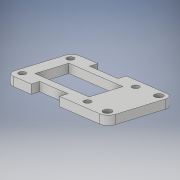
# Autodesk Inventor part: 板子6
Saved by Autodesk Inventor 2017 (Build 210142000, 142)
## iProperties
Part Number: 板子6
Material: 一般
Document SubType Name: Modeling
Designer: User
Density: 1 g/cm^3
Appearance: 預設
Author: User
Autodesk Inventor part; units mm, degrees
ref_plane "YZ Plane" through (0, 0, 0) normal (1, 0, 0) x (0, 1, 0)
ref_plane "XZ Plane" through (0, 0, 0) normal (0, 1, 0) x (-1, 0, 0)
ref_plane "XY Plane" through (0, 0, 0) normal (0, 0, 1) x (1, 0, 0)
sketch "草圖1" plane through (0, 0, 0) normal (0, 1, 0) x (-1, 0, 0)
  line L0 (-21.25, 11.85) -> (-21.25, -11.85)
  line L1 (-21.25, -11.85) -> (21.25, -11.85)
  line L2 (21.25, -11.85) -> (21.25, 11.85)
  line L3 (0, -16.59) -> (0, 16.59) projected
  line L4 (29.75, 0) -> (-29.75, 0) projected
  circle A0 centre (18.45, 8.55) radius 1.25
  circle A1 centre (18.45, -8.55) radius 1.25
  line L5 (16.05, 6) -> (-6.75, 6)
  line L6 (-6.75, 6) -> (-6.75, -6)
  line L7 (-6.75, -6) -> (16.05, -6)
  line L8 (16.05, -6) -> (16.05, 6)
  line L9 (10.75, -11.85) -> (-1.25, -11.85)
  line L10 (-1.25, -11.85) -> (-1.25, -8.85)
  line L11 (-1.25, -8.85) -> (10.75, -8.85)
  line L12 (10.75, -8.85) -> (10.75, -11.85)
  line L13 (16.05, -6) -> (4.65, -6)
  line L14 (4.65, -6) -> (4.65, 4.0143)
  circle A2 centre (-9.15, 8.55) radius 1.25
  circle A3 centre (-9.15, -8.55) radius 1.25
  line L15 (-1.25, 11.85) -> (-1.25, 8.85)
  line L16 (-1.25, 8.85) -> (10.75, 8.85)
  line L17 (10.75, 8.85) -> (10.75, 11.85)
  circle A4 centre (-18.25, 9.1) radius 1.5
  circle A5 centre (-18.25, -9.1) radius 1.5
  line L18 (21.25, 11.85) -> (10.75, 11.85)
  line L19 (-1.25, 11.85) -> (-21.25, 11.85)
  point P0 (0, 0)
  point P1 (0, 0)
  dimension "d12" = 23.7
  dimension "d13" = 42.5
  dimension "d14" = 2.8
  dimension "d15" = 2.5
  dimension "d17" = 5.2
  dimension "d20" = 12
  dimension "d21" = 6
  dimension "d22" = 22.8
  dimension "d23" = 10.5
  dimension "d24" = 3
  dimension "d25" = 12
  dimension "d26" = 11.4
  dimension "d27" = 3
  dimension "d28" = 3
  dimension "d30" = 3
  dimension "d31" = 2.75
  dimension "d32" = 3
  constraints: 36 end point, 7 parallel, 7 symmetric about line, 6 centre point, 5 perpendicular, 4 horizontal, 1 midpoint, 1 point on line, 4 other
  measures "d12" distance of L1.end L2.end
  measures "d13" distance of L0.end L1.end
  measures "d14" distance from line of L2 A0.centre
  measures "d15" diameter of A0
  measures "d17" distance between parallel lines of L8 L2
  measures "d20" distance of L7.end L5.start
  measures "d21" distance between parallel lines of L4 L7
  measures "d22" distance of L6.end L7.end
  measures "d23" distance between parallel lines of L2 L12
  measures "d24" distance of L11.end L9.start
  measures "d25" distance of L10.end L11.end
  measures "d26" distance of L7.end L13.end
  measures "d27" diameter of A4
  measures "d28" diameter of A5
  measures "d30" distance from line of L0 A4.centre
  measures "d31" distance from line of L1 A5.centre
  measures "d32" distance from line of L0 A5.centre
extrude "擠出1" add sketch "草圖1" along normal mid plane 3 contours L19 L15 L16 L3 L5 L6 L4 L0 | L4 L6 L7 L3 L11 L10 L1 L0 | L16 L17 L18 L2 L4 L8 L5 L3 | L7 L8 L4 L2 L1 L12 L11 L3
fillet "圓角1" radius 3 4 edges at (-21.25, 0, 11.85) (-21.25, 0, -11.85) (21.25, 0, 11.85) (21.25, 0, -11.85)
